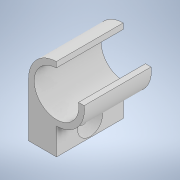
# Autodesk Inventor part: shadeHolderV02
Saved by Autodesk Inventor 2021.2 (Build 252289000, 289)
## iProperties
Created: 2021-02-12
Part Number: shadeHolderV02
Material: Generic
Document SubType Name: Modeling
Designer: robst
Density: 1 g/cm^3
Appearance: Default
Author: robst
Autodesk Inventor part; units mm, degrees
ref_plane "YZ Plane" through (0, 0, 0) normal (1, 0, 0) x (0, 1, 0)
ref_plane "XZ Plane" through (0, 0, 0) normal (0, 1, 0) x (-1, 0, 0)
ref_plane "XY Plane" through (0, 0, 0) normal (0, 0, 1) x (1, 0, 0)
sketch "Sketch4" plane through (0, 0, 0) normal (0, 0, 1) x (1, 0, 0)
  arc A0 (-0.06, 6.3497) -> (6.2637, 1.0435) centre (0, 0) ccw
  arc A1 (-1.7259, 7.7476) -> (7.9296, -0.3544) centre (0, 0) ccw
  line L0 (0, 0) -> (0, 7.9375) construction
  line L1 (-0.06, 6.3497) -> (6.2637, 1.0435) construction
  line L2 (-0.06, 6.3497) -> (-1.7259, 7.7476)
  line L3 (6.2637, 1.0435) -> (7.9296, -0.3544)
  circle A2 centre (0, 0) radius 6.35
  dimension "d10" = 12.7
  dimension "d11" = 1.5875
  dimension "d12" = 50
  dimension "d13" = 8.255
  constraints: 8 end point, 4 point on circle, 3 centre point, 3 coincident, 1 collinear, 1 concentric, 1 point on line, 1 vertical
  measures "d10" diameter of A0
  measures "d11" radial gap between concentric circles of A1 A0
  measures "d12" angle of L1 L0
  measures "d13" distance of L1.start L1.end
extrude "Extrusion3" add sketch "Sketch4" along normal mid plane 19.05 contours A0 L3 A1 L2
sketch "Sketch5" plane through (0, 0, 0) normal (0, 0, 1) x (1, 0, 0)
  arc A0 (-1.7259, 7.7476) -> (7.9296, -0.3544) centre (0, 0) ccw projected
  line L0 (-7.9375, 0) -> (-7.9375, -15.5575)
  line L1 (-7.9375, -15.5575) -> (0, -15.5575)
  line L2 (0, -15.5575) -> (0, -7.9375)
  circle A1 centre (0, 0) radius 7.9375
  dimension "d16" = 7.62
  constraints: 6 end point, 2 perpendicular, 2 point on circle, 1 centre point, 1 coincident, 1 tangent, 1 vertical
  measures "d16" distance from line of L2.end L1
extrude "Extrusion4" add sketch "Sketch5" along normal mid plane 19.05 contours A0 L2 L1 L0
sketch "Sketch6" plane through (0, -15.5575, 9.525) normal (1, 0, 0) x (0, 0, -1)
  line L0 (0, 7.62) -> (19.05, 7.62) projected
  line L1 (19.05, 7.62) -> (19.05, 0) projected
  line L2 (0, 0) -> (19.05, 0) projected
  line L3 (0, 0) -> (0, 7.62) projected
  line L4 (0, 7.62) -> (19.05, 0) construction
  line L5 (19.05, 7.62) -> (0, 0) construction
  point P0 (9.525, 15.5575)
  point P1 (9.525, 3.81)
  constraints: 4 end point, 1 midpoint
hole "Hole1" at (0, -11.7475, 0) direction (-1, 0, 0) diameter 3.5052 end through all countersink diameter 7.112 countersink angle 82
sketch "Sketch7" plane through (0, 0, 0) normal (0, 0, 1) x (1, 0, 0)
  arc A0 (-0.06, 6.3497) -> (6.2637, 1.0435) centre (0, 0) ccw projected
  arc A1 (-1.7259, 7.7476) -> (-7.9375, 0) centre (0, 0) ccw projected
  line L0 (-0.06, 6.3497) -> (-1.7259, 7.7476) projected
  line L1 (7.9296, -0.3544) -> (6.2637, 1.0435) projected
  arc A2 (0, -7.9375) -> (7.9296, -0.3544) centre (0, 0) ccw projected
  line L2 (-0.06, 6.3497) -> (-0.06, 7.9373)
  line L3 (6.2637, 1.0435) -> (7.8686, 1.0435)
  line L4 (6.2637, 1.0435) -> (7.9296, -0.3544)
  arc A3 (-0.06, 7.9373) -> (-1.7259, 7.7476) centre (0, 0) ccw
  arc A4 (7.9296, -0.3544) -> (7.8686, 1.0435) centre (0, 0) ccw
  constraints: 7 end point, 4 point on circle, 2 centre point, 1 collinear, 1 perpendicular, 1 vertical
extrude "FillInCornerPieces" add sketch "Sketch7" along normal mid plane 19.05
equation "\"d10\" = shadeDiameter"
equation "\"d11\" = shadeHolderWallThickness"
equation "\"d14\" = partWidth"
equation "\"d16\" = flatBelowShade"
equation "\"d17\" = partWidth"
equation "\"d26\" = partWidth"
equation "\"shadeDiameter\" = 12.7"
equation "\"partWidth\" = 19.05"
equation "\"backThickness\" = 1.905"
equation "\"backHeight\" = 25.4"
equation "\"cutTiltAngle\" = 40deg"
equation "\"flatBelowShade\" = 7.62"
equation "\"shadeHolderWallThickness\" = 1.5875"
body "Solid2"
